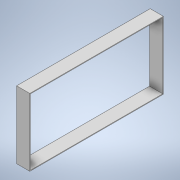
# Autodesk Inventor part: vib_bed_full_yz
Saved by Autodesk Inventor 2021 (Build 250183000, 183)
## iProperties
Created: 2020-07-18
Part Number: vib_bed_full_yz
Material: Generic
Document SubType Name: Modeling
Designer: dwer2
Density: 1 g/cm^3
Appearance: Default
Author: dwer2
Autodesk Inventor part; units mm, degrees
ref_plane "YZ Plane" through (0, 0, 0) normal (1, 0, 0) x (0, 1, 0)
ref_plane "XZ Plane" through (0, 0, 0) normal (0, 1, 0) x (-1, 0, 0)
ref_plane "XY Plane" through (0, 0, 0) normal (0, 0, 1) x (1, 0, 0)
sketch "Sketch1" plane through (0, 0, 0) normal (1, 0, 0) x (0, 1, 0)
  line L0 (0, 0) -> (100, 0)
  line L1 (100, 0) -> (100, 200)
  line L2 (100, 200) -> (0, 200)
  line L3 (0, 200) -> (0, 0)
  line L4 (-1, 201) -> (101, 201)
  line L5 (101, 201) -> (101, -1)
  line L6 (101, -1) -> (-1, -1)
  line L7 (-1, -1) -> (-1, 201)
  dimension "inner_width" = 100
  dimension "height" = 200
  dimension "wall_thicknes" = 1
  dimension "d3" = 1
  dimension "d4" = 1
  dimension "d5" = 1
  constraints: 16 end point, 4 parallel, 2 horizontal, 2 perpendicular
  measures "inner_width" distance of L1.end L2.end
  measures "height" distance of L0.end L1.end
  measures "wall_thicknes" distance between parallel lines of L1 L5
  measures "d3" distance between parallel lines of L3 L7
  measures "d4" distance between parallel lines of L0 L6
  measures "d5" distance between parallel lines of L4 L2
extrude "Extrusion1" add sketch "Sketch1" along normal blind 20
equation "\"d3\" = wall_thicknes"
equation "\"d4\" = wall_thicknes"
equation "\"d5\" = wall_thicknes"
body "Solid1"
